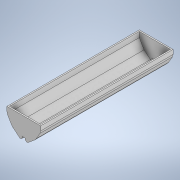
# Autodesk Inventor part: ModelProfil1
Saved by Autodesk Inventor 2020.3 (Build 243373000, 373)
## iProperties
Created: 2021-03-14
Part Number: ModelProfil1
Material: Generic
Document SubType Name: Modeling
Designer: alexo
Density: 1 g/cm^3
Appearance: Default
Author: alexo
Autodesk Inventor part; units mm, degrees
ref_plane "YZ Plane" through (0, 0, 0) normal (1, 0, 0) x (0, 1, 0)
ref_plane "XZ Plane" through (0, 0, 0) normal (0, 1, 0) x (-1, 0, 0)
ref_plane "XY Plane" through (0, 0, 0) normal (0, 0, 1) x (1, 0, 0)
sketch "Sketch1" plane through (0, 0, 0) normal (0, 0, 1) x (1, 0, 0)
  line L0 (0, 9.1429) -> (0, -9.1429) construction
  line L1 (0, -7.1429) -> (-1, -7.1429)
  line L2 (-1, -7.1429) -> (-1, -9.1429)
  line L3 (-1, -9.1429) -> (-3, -9.1429)
  line L4 (-3, -9.1429) -> (-8.9507, -4.1496)
  line L5 (-8.9507, -4.1496) -> (-12.7556, 2.4407)
  line L6 (-12.7556, 2.4407) -> (-12.7556, 6.7581)
  line L7 (-12.7556, 6.7581) -> (0, 6.7581)
  line L8 (0, -7.1429) -> (1, -7.1429)
  line L9 (1, -7.1429) -> (1, -9.1429)
  line L10 (1, -9.1429) -> (3, -9.1429)
  line L11 (3, -9.1429) -> (8.9507, -4.1496)
  line L12 (8.9507, -4.1496) -> (12.7556, 2.4407)
  line L13 (12.7556, 2.4407) -> (12.7556, 6.7581)
  line L14 (12.7556, 6.7581) -> (0, 6.7581)
  point P0 (0, 0)
  point P1 (0, 0)
  dimension "d0" = 2
  dimension "d1" = 2
  dimension "d2" = 1
  dimension "d3" = 160
  dimension "d4" = 150
  constraints: 30 end point, 6 symmetric about line, 3 perpendicular, 2 point on line, 1 coincident, 1 horizontal, 1 midpoint, 1 parallel, 1 vertical
  measures "d0" distance of L1.end L2.end
  measures "d1" distance of L2.end L3.end
  measures "d2" distance of L1.start L1.end
  measures "d3" angle of L4 L5
  measures "d4" angle of L5 L6
extrude "Extrusion1" add sketch "Sketch1" along normal blind 100
shell "Shell1" thickness 1 removed faces 2 at (-4.2519, 6.7581, 66.6667) at (8.5037, 6.7581, 33.3333)
chamfer "Chamfer1" distance 1 angle 45 6 edges at (1, -9.1429, 50) (-1, -9.1429, 50) (8.9507, -4.1496, 50) (12.7556, 2.4407, 50) (-8.9507, -4.1496, 50) (-12.7556, 2.4407, 50)
body "Solid1"
